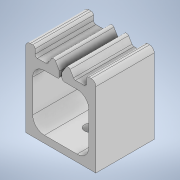
# Autodesk Inventor part: Cable Holder
Saved by Autodesk Inventor 2022 (Build 260153000, 153)
## iProperties
Created: 2022-03-20
Part Number: Cable Holder
Material: Generic
Document SubType Name: Modeling
Designer: torba
Density: 1 g/cm^3
Appearance: Default
Author: torba
Autodesk Inventor part; units mm, degrees
ref_plane "YZ Plane" through (0, 0, 0) normal (1, 0, 0) x (0, 1, 0)
ref_plane "XZ Plane" through (0, 0, 0) normal (0, 1, 0) x (-1, 0, 0)
sketch "Sketch3" plane through (0, 0, 0) normal (0, 0, 1) x (1, 0, 0)
  line L0 (0, 0) -> (30, 0)
  line L1 (30, 0) -> (30, 30)
  line L2 (30, 30) -> (0, 30)
  line L3 (0, 30) -> (0, 0)
  line L4 (3, 3) -> (27, 3)
  line L5 (27, 3) -> (27, 27)
  line L6 (27, 27) -> (3, 27)
  line L7 (3, 27) -> (3, 3)
  dimension "d8" = 30
  dimension "d9" = 30
  dimension "d10" = 3
  constraints: 16 end point, 4 parallel, 2 perpendicular, 1 horizontal, 3 other
  measures "d8" distance of L2.end L1.end
  measures "d9" distance of L1.end L0.end
  measures "d10" distance between parallel lines of L3 L7
extrude "Extrusion2" add sketch "Sketch3" along normal blind 25
fillet "Fillet1" radius 5 2 edges at (3, 3, 12.5) (27, 3, 12.5)
fillet "Fillet2" radius 5 2 edges at (3, 27, 12.5) (27, 27, 12.5)
sketch "Sketch4" plane through (0, 0, 25) normal (0, 0, 1) x (1, 0, 0)
  line L0 (30, 30) -> (0, 30) projected
  line L1 (0, 30) -> (0, 0) projected
  line L2 (0, 0) -> (30, 0) projected
  line L3 (30, 0) -> (30, 30) projected
  line L4 (3, 8) -> (3, 22) projected
  arc A0 (8, 27) -> (3, 22) centre (8, 22) ccw projected
  line L5 (8, 27) -> (22, 27) projected
  arc A1 (27, 22) -> (22, 27) centre (22, 22) ccw projected
  line L6 (27, 22) -> (27, 8) projected
  arc A2 (22, 3) -> (27, 8) centre (22, 8) ccw projected
  line L7 (22, 3) -> (8, 3) projected
  arc A3 (3, 8) -> (8, 3) centre (8, 8) ccw projected
  line L8 (25, 30) -> (5, 30) projected
  line L9 (15, 30) -> (15, 27)
  line L10 (8, 27) -> (22, 27) projected
  line L11 (14.5, 27) -> (15.5, 27)
  line L12 (15.5, 27) -> (15.5, 30)
  line L13 (15.5, 30) -> (14.5, 30)
  line L14 (14.5, 30) -> (14.5, 27)
  line L15 (14.5, 27) -> (15.5, 30) construction
  line L16 (15.5, 27) -> (14.5, 30) construction
  point P0 (15, 28.5)
  dimension "d15" = 1
  constraints: 14 end point, 5 midpoint, 2 parallel, 1 horizontal, 1 perpendicular, 1 point on line
  measures "d15" distance of L13.end L12.end
extrude "Extrusion3" cut sketch "Sketch4" against normal blind 25 contours L12 L5 L9 L0 | L9 L5 L14 L0
sketch "Sketch5" plane through (0, 0, 25) normal (0, 0, 1) x (1, 0, 0)
  line L0 (22, 3) -> (8, 3) projected
  line L1 (15, 3) -> (15, 43.6713) construction
  line L2 (14.5, 27) -> (14.5, 30) projected
  line L3 (14.5, 30) -> (9.5, 30)
  line L4 (14.5, 30) -> (15.5, 30) projected
  line L5 (14.5, 30) -> (11.8684, 34.2514)
  line L6 (15.5, 30) -> (15.5, 27) projected
  line L7 (15.5, 27) -> (22, 27) projected
  arc A0 (27, 22) -> (22, 27) centre (22, 22) ccw projected
  line L8 (27, 22) -> (27, 8) projected
  arc A1 (22, 3) -> (27, 8) centre (22, 8) ccw projected
  line L9 (22, 3) -> (8, 3) projected
  arc A2 (3, 8) -> (8, 3) centre (8, 8) ccw projected
  line L10 (3, 8) -> (3, 22) projected
  arc A3 (8, 27) -> (3, 22) centre (8, 22) ccw projected
  line L11 (8, 27) -> (14.5, 27) projected
  line L12 (14.5, 27) -> (14.5, 30) projected
  line L13 (14.5, 30) -> (0, 30) projected
  line L14 (0, 30) -> (0, 0) projected
  line L15 (0, 0) -> (30, 0) projected
  line L16 (30, 0) -> (30, 30) projected
  line L17 (30, 30) -> (15.5, 30) projected
  line L18 (11.8684, 34.2514) -> (9.2368, 30)
  line L19 (14.5, 30) -> (0, 30) projected
  line L20 (0, 30) -> (0, 0) projected
  line L21 (0, 30) -> (4, 30)
  line L22 (4, 30) -> (4, 34)
  line L23 (4, 34) -> (0, 34)
  line L24 (0, 34) -> (0, 30)
  dimension "d18" = 5
  dimension "d19" = 5
  dimension "d27" = 5
  dimension "d28" = 58.243
  dimension "d29" = 13.6713
  dimension "d30" = 4
  dimension "d31" = 4
  constraints: 16 end point, 2 parallel, 2 point on line, 1 horizontal, 1 midpoint, 1 perpendicular, 1 vertical
  measures "d18" distance of L2.end L3.end
  measures "d19" distance of L2.end L5.end
  measures "d27" distance of L5.end L18.end
  measures "d28" angle of L9 L5
  measures "d29" distance from line of L1.end L4
  measures "d30" distance of L23.end L22.end
  measures "d31" distance of L22.end L21.end
extrude "Extrusion4" add sketch "Sketch5" against normal up to surface (25 mm away) contours L3 L13 L18 L5 | L13 L24 L23 L22
fillet "Fillet5" radius 2 1 edges at (0, 34, 12.5)
fillet "Fillet6" radius 1 2 edges at (4, 34, 12.5) (11.8684, 34.2514, 12.5)
ref_plane "Work Plane2" through (15, 0, 0) normal (-1, 0, 0) x (0, 0, 1)
mirror "Mirror1" about plane through (15, 0, 0) normal (-1, 0, 0) of "Extrusion4", "Fillet5", "Fillet6"
sketch "Sketch7" plane through (8, 3, 0) normal (0, 1, 0) x (1, 0, 0)
  line L0 (-8, 0) -> (0, 0) projected
  line L1 (0, 0) -> (14, 0) projected
  line L2 (14, 0) -> (22, 0) projected
  line L3 (22, 0) -> (22, -25) projected
  line L4 (22, -25) -> (14, -25) projected
  line L5 (14, -25) -> (14, 0) projected
  line L6 (-8, -25) -> (-8, 0) projected
  line L7 (0, -25) -> (-8, -25) projected
  line L8 (14, -25) -> (0, -25) projected
  line L9 (0, -25) -> (0, 0) projected
  line L10 (0, 0) -> (14, -25)
  circle A0 centre (7, -12.5) radius 2.3812
  dimension "d34" = 4.7625
  constraints: 2 end point, 1 centre point, 1 midpoint
  measures "d34" diameter of A0
extrude "Extrusion6" cut sketch "Sketch7" against normal blind 10 contours A0 L10 | L10 A0
fillet "Fillet3" radius 1 6 edges at (14.5, 27, 12.5) (15.5, 27, 12.5) (9.2368, 30, 12.5) (20.7632, 30, 12.5) (4, 30, 12.5) (26, 30, 12.5)
body "Solid2"
